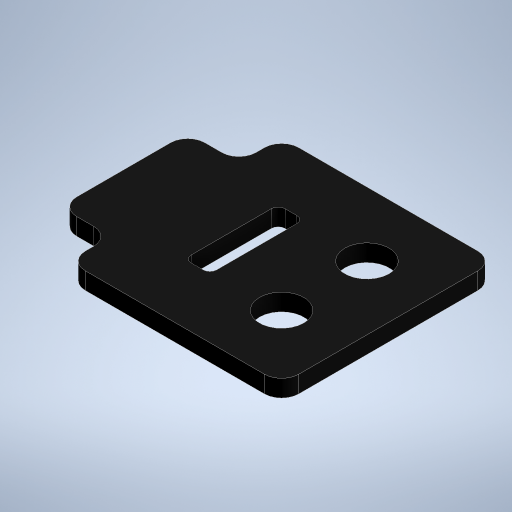
# Autodesk Inventor part: pokrywka
Saved by Autodesk Inventor 2024.2 (Build 282272000, 272)
## iProperties
Created: 2024-01-16
Part Number: pokrywka
Material: PLA
Document SubType Name: Modeling
Designer: Konrad
Density: 1 g/cm^3
Appearance: PLA
Author: Konrad
Autodesk Inventor part; units mm, degrees
ref_plane "YZ Plane" through (0, 0, 0) normal (1, 0, 0) x (0, 1, 0)
ref_plane "XZ Plane" through (0, 0, 0) normal (0, 1, 0) x (-1, 0, 0)
ref_plane "XY Plane" through (0, 0, 0) normal (0, 0, 1) x (1, 0, 0)
sketch "Szkic1" plane through (0, 0, 0) normal (0, 1, 0) x (-1, 0, 0)
  line L0 (0, 0) -> (25, 0)
  line L1 (25, 0) -> (25, -25)
  line L2 (25, -25) -> (0, -25)
  line L3 (0, -25) -> (0, 0)
  line L4 (25, -5) -> (31, -5)
  line L5 (31, -5) -> (31, -20)
  line L6 (31, -20) -> (25, -20)
  line L7 (25, -20) -> (25, -5)
  circle A0 centre (7.5, -7.5) radius 2.6
  circle A1 centre (7.5, -17.5) radius 2.6
  line L8 (25, -12.5) -> (0, -12.5) construction
  line L9 (18.4, -18) -> (15.4, -18)
  line L10 (15.4, -18) -> (15.4, -7)
  line L11 (15.4, -7) -> (18.4, -7)
  line L12 (18.4, -7) -> (18.4, -18)
  dimension "d0" = 5.2
  dimension "d1" = 25
  dimension "d2" = 25
  dimension "d3" = 7.5
  dimension "d4" = 10
  dimension "d5" = 6
  dimension "d6" = 15
  dimension "d10" = 18.4
  dimension "d11" = 11
  dimension "d12" = 3
  constraints: 26 end point, 6 parallel, 3 horizontal, 3 perpendicular, 2 centre point, 2 midpoint, 1 equal radius, 1 point on line, 1 symmetric about line, 2 other
  measures "d0" diameter of A0
  measures "d1" distance between parallel lines of L2 L0
  measures "d2" distance of L1.end L2.end
  measures "d3" distance from line of L3 A0.centre
  measures "d4" distance of A1.centre A0.centre
  measures "d5" distance of L5.end L6.end
  measures "d6" distance of L4.end L5.end
  measures "d10" distance between parallel lines of L3 L12
  measures "d11" distance of L11.end L9.start
  measures "d12" distance of L9.start L9.end
extrude "Wyciągnięcie proste1" add sketch "Szkic1" along normal blind 2
fillet "Zaokrąglenie1" radius 2 8 edges at (0, 1, 0) (0, 1, -25) (-25, 1, 0) (-25, 1, -5) (-31, 1, -5) (-31, 1, -20) (-25, 1, -20) (-25, 1, -25)
fillet "Zaokrąglenie2" radius 0.8 4 edges at (-18.4, 1, -18) (-15.4, 1, -18) (-18.4, 1, -7) (-15.4, 1, -7)
